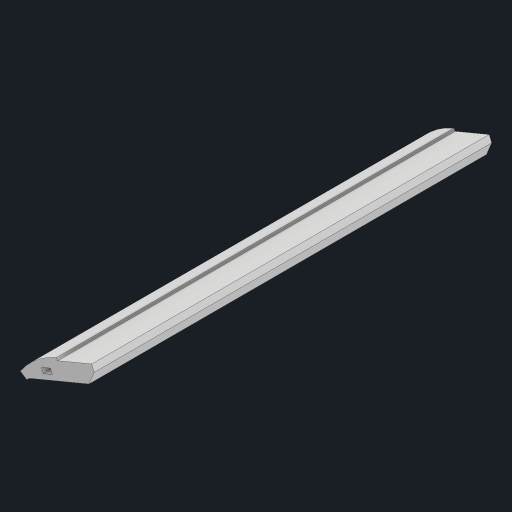
# Autodesk Inventor part: ESQUINA_REDONDEADA_R50
Saved by Autodesk Inventor 2024.3 (Build 283343000, 343)
## iProperties
Created: 2024-05-19
Part Number: ESQUINA_REDONDEADA_R50
Material: Generic
Document SubType Name: Modeling
Designer: Niler
Density: 1 g/cm^3
Appearance: Default
Author: Niler
Autodesk Inventor part; units mm, degrees
ref_plane "YZ Plane" through (0, 0, 0) normal (1, 0, 0) x (0, 1, 0)
ref_plane "XZ Plane" through (0, 0, 0) normal (0, 1, 0) x (-1, 0, 0)
ref_plane "XY Plane" through (0, 0, 0) normal (0, 0, 1) x (1, 0, 0)
sketch "Sketch1" plane through (0, 0, 0) normal (0, 0, 1) x (1, 0, 0)
  line L0 (10, 0) -> (-1.5, 0) projected
  line L1 (10, 45.2667) -> (10, 0) projected
  arc A0 (13.0769, 49.8821) -> (10, 45.2667) centre (15, 45.2667) ccw projected
  line L2 (54.8615, 67.2923) -> (13.0769, 49.8821) projected
  line L3 (50.4385, 77.9077) -> (54.8615, 67.2923) projected
  line L4 (50.4385, 77.9077) -> (29.2692, 69.0872) projected
  arc A1 (29.2692, 69.0872) -> (-1.5, 22.9333) centre (48.5, 22.9333) ccw projected
  line L5 (-1.5, 0) -> (-1.5, 22.9333) projected
  line L6 (29.2692, 69.0872) -> (33.9692, 58.5872)
  line L7 (15, 45.2667) -> (6.8975, 50.6683)
  line L8 (29.2692, 69.0872) -> (50.4077, 77.8949)
  line L9 (50.4077, 77.8949) -> (52.5231, 72.8179)
  line L10 (52.5231, 72.8179) -> (49.2923, 64.9718)
  line L11 (29.8823, 67.7176) -> (50.9846, 76.5103)
  point P0 (0, 0)
  point P1 (10.8397, 48.0402)
  dimension "d2" = 22.9
  dimension "d3" = 5.5
  dimension "d4" = 45
  dimension "d5" = 1.5
  constraints: 12 end point, 4 point on line, 1 midpoint, 1 parallel, 1 perpendicular, 1 point on circle, 1 tangent
  measures "d2" distance of L4.end L8.end
  measures "d3" distance of L8.end L9.end
  measures "d4" angle of L2 L10
  measures "d5" distance between parallel lines of L8 L11
extrude "Extrusion1" add sketch "Sketch1" along normal blind 245.5 contours L7 A1 L6 L2 A0 | L6 L11 L9 L10 L2
sketch "Sketch2" plane through (10.8397, 48.0402, 0) normal (-0.5547002, -0.8320503, 0) x (0.8320503, -0.5547002, 0)
  line L0 (-4.738, 0) -> (0, 0) projected
  line L1 (0, 0) -> (0, 245.5) projected
  line L2 (-4.738, 245.5) -> (0, 245.5) projected
  line L3 (-4.738, 0) -> (-4.738, 245.5) projected
  circle A0 centre (-2.238, 15) radius 1.25
  circle A1 centre (-2.238, 65) radius 1.25
  circle A2 centre (-2.238, 115) radius 1.25
  circle A3 centre (-2.238, 165) radius 1.25
  circle A4 centre (-2.238, 215) radius 1.25
  point P0 (17.6287, 0)
  dimension "d6" = 2.5
  dimension "d7" = 2.5
  dimension "d8" = 15
  dimension "d11" = 50
  constraints: 5 centre point, 1 vertical, 8 other
  measures "d6" diameter of A0
  measures "d7" distance from line of L3 A0.centre
  measures "d8" distance from line of L0 A0.centre
  measures "d11" distance of A0.centre A1.centre
extrude "Extrusion2" cut sketch "Sketch2" against normal blind 3 contours A0 | A1 | A2 | A3 | A4
sketch "Sketch3" plane through (0, 0, 0) normal (0, 0, -1) x (-1, 0, 0)
  line L0 (-13.0769, 49.8821) -> (-49.2923, 64.9718) projected
  line L1 (-26.6245, 58.7769) -> (-21.086, 56.4692)
  line L2 (-21.086, 56.4692) -> (-19.9322, 59.2384)
  line L3 (-19.9322, 59.2384) -> (-25.4706, 61.5461)
  line L4 (-25.4706, 61.5461) -> (-26.6245, 58.7769)
  arc A0 (-10.8397, 48.0402) -> (-13.0769, 49.8821) centre (-15, 45.2667) ccw projected
  line L5 (-6.8975, 50.6683) -> (-10.8397, 48.0402) projected
  arc A1 (-6.8975, 50.6683) -> (-29.2692, 69.0872) centre (-48.5, 22.9333) ccw projected
  line L6 (-29.8823, 67.7176) -> (-29.2692, 69.0872) projected
  line L7 (-50.9846, 76.5103) -> (-29.8823, 67.7176) projected
  line L8 (-52.5231, 72.8179) -> (-50.9846, 76.5103) projected
  line L9 (-49.2923, 64.9718) -> (-52.5231, 72.8179) projected
  line L10 (-13.0769, 49.8821) -> (-49.2923, 64.9718) projected
  point P0 (0, 0)
  dimension "d20" = 6
  dimension "d21" = 3
  dimension "d22" = 3
  dimension "d32" = 12.7
  constraints: 8 end point, 2 parallel, 2 perpendicular
  measures "d20" distance of L1.start L1.end
  measures "d21" distance of L3.end L1.start
  measures "d22" distance between parallel lines of L0 L1
  measures "d32" distance from line of L2 L5.end
extrude "Extrusion3" cut sketch "Sketch3" against normal blind 30 contours L4 L3 L2 L1
sketch "Sketch4" plane through (49.2923, 64.9718, 0) normal (0.3846154, -0.9230769, 0) x (0.9230769, 0.3846154, 0)
  line L0 (-29.3068, 0) -> (-23.3068, 0) projected
  line L1 (-29.3068, 0) -> (-29.3068, 30) projected
  line L2 (-29.3068, 30) -> (-23.3068, 30) projected
  line L3 (-23.3068, 0) -> (-23.3068, 30) projected
  circle A0 centre (-26.3068, 26.4) radius 1.65
  line L4 (-26.3068, 29.7486) -> (-23.4068, 28.0743)
  line L5 (-23.4068, 28.0743) -> (-23.4068, 24.7257)
  line L6 (-23.4068, 24.7257) -> (-26.3068, 23.0514)
  line L7 (-26.3068, 23.0514) -> (-29.2068, 24.7257)
  line L8 (-29.2068, 24.7257) -> (-29.2068, 28.0743)
  line L9 (-29.2068, 28.0743) -> (-26.3068, 29.7486)
  point P0 (-70.4897, 0)
  point P1 (-26.3068, 30)
  dimension "d26" = 3.3
  dimension "d27" = 3.6
  dimension "d28" = 5.8
  constraints: 12 end point, 2 vertical alignment, 1 centre point, 1 coincident, 1 midpoint, 13 other
  measures "d26" diameter of A0
  measures "d27" distance from line of L2 A0.centre
  measures "d28" distance between parallel lines of L5 L8
extrude "Extrusion4" cut sketch "Sketch4" against normal blind 7 contours A0
ref_plane "Work Plane1" through (0, 0, 122.75) normal (0, 0, -1) x (-1, 0, 0)
mirror "Mirror1" about plane through (0, 0, 122.75) normal (0, 0, -1) of "Extrusion4", "Extrusion3"
body "Solid1"
